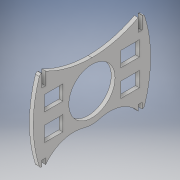
# Autodesk Inventor part: Cuerpo - Unión Laterales
Saved by Autodesk Inventor 2019 (Build 230136000, 136)
## iProperties
Created: 2020-02-15
Part Number: Cuerpo - Unión Laterales
Material: Genérico
Document SubType Name: Chapa
Designer: Mafer1
Density: 1 g/cm^3
Appearance: Valor por defecto
Sheet Metal Rule: Default
Mass: 19.1194 g
Surface Area: 143.282 cm^2
Volume: 19.1194 cm^3
soporte: 60.000 mm
largo_base: 200.000 mm
ancho_base: 80.000 mm
Author: Mafer1
Autodesk Inventor part; units mm, degrees
ref_plane "YZ Plane" through (0, 0, 0) normal (1, 0, 0) x (0, 1, 0)
ref_plane "XZ Plane" through (0, 0, 0) normal (0, 1, 0) x (-1, 0, 0)
ref_plane "XY Plane" through (0, 0, 0) normal (0, 0, 1) x (1, 0, 0)
sketch "Boceto1" plane through (0, 0, 0) normal (1, 0, 0) x (0, 1, 0)
  circle A0 centre (0, 0) radius 25
  line L0 (35, 43.5516) -> (35, 40)
  line L1 (-35, 43.5516) -> (-35, 40)
  line L2 (35, -40) -> (35, -43.5516)
  line L3 (-35, -40) -> (-35, -43.5516)
  arc A1 (33.6111, 45.4559) -> (-33.6111, 45.4559) centre (0, -59.2833) ccw
  arc A2 (-33.6111, -45.4559) -> (33.6111, -45.4559) centre (0, 59.2833) ccw
  arc A3 (-24.0379, 6.8686) -> (-35, 40) centre (-53.845, 15.3856) ccw
  arc A4 (-35, -40) -> (-24.0379, -6.8686) centre (-53.845, -15.3856) ccw
  arc A5 (35, 40) -> (24.9998, -0.1114) centre (111.9989, -0.499) ccw
  arc A6 (24.9998, 0.1114) -> (35, -40) centre (111.9989, 0.499) ccw
  arc A7 (35, 43.5516) -> (33.6111, 45.4559) centre (33, 43.5516) ccw
  arc A8 (-33.6111, 45.4559) -> (-35, 43.5516) centre (-33, 43.5516) ccw
  arc A9 (33.6111, -45.4559) -> (35, -43.5516) centre (33, -43.5516) ccw
  arc A10 (-35, -43.5516) -> (-33.6111, -45.4559) centre (-33, -43.5516) ccw
  point P0 (35, 45)
  point P1 (-35, 45)
  point P2 (35, -45)
  point P3 (-35, -45)
  dimension "d0" = 50
  dimension "d1" = 5
  dimension "d2" = 70
  dimension "d3" = 35
  dimension "d4" = 0
  dimension "d5" = 70
  dimension "d6" = 0
  dimension "d8" = 40
  dimension "d9" = 40
  dimension "d10" = 110
  dimension "d12" = 110
  dimension "d13" = 31
  dimension "d14" = 31
  dimension "d15" = 87
  dimension "d17" = 87
  dimension "d20" = 2
  dimension "d21" = 2
  dimension "d22" = 2
  constraints: 28 point on circle, 12 tangent, 11 centre point, 8 end point, 4 point on line, 4 vertical, 3 equal length, 1 coincident, 1 collinear, 1 equal radius
  measures "d0" diameter of A0
  measures "d1" distance of point (35, 45) L0.end
  measures "d2" distance between parallel lines of L1 L0
  measures "d3" distance from line of L1 point (0, 0)
  measures "d4" vertical distance of point (-35, 45) point (35, 45)
  measures "d5" distance between parallel lines of L3 L2
  measures "d6" vertical distance of point (-35, -45) point (35, -45)
  measures "d8" vertical distance of point (0, 0) L0.end
  measures "d9" vertical distance of L2.start point (0, 0)
  measures "d10" radius of A1
  measures "d12" radius of A2
  measures "d13" radius of A3
  measures "d14" radius of A4
  measures "d15" radius of A5
  measures "d17" radius of A6
  measures "d20" radius of A7
  measures "d21" radius of A9
  measures "d22" radius of A10
extrude "Extrusión1" add sketch "Boceto1" along normal blind 3.3
sketch "Boceto2" plane through (3.3, 0, 0) normal (1, 0, 0) x (0, 0, -1)
  arc A0 (-40, 35) -> (0, 25.0003) centre (0.499, 111.9989) ccw projected
  arc A1 (40, -35) -> (6.8686, -24.0379) centre (15.3856, -53.845) ccw projected
  arc A2 (0, 25.0003) -> (40, 35) centre (-0.499, 111.9989) ccw projected
  arc A3 (-6.8686, -24.0379) -> (-40, -35) centre (-15.3856, -53.845) ccw projected
  line L0 (-40, 35) -> (-43.3, 35)
  line L1 (-43.3, 35) -> (-43.3, 24)
  line L2 (-43.3, 24) -> (-40, 24)
  line L3 (-40, 24) -> (-40, 35)
  line L4 (-40, -35) -> (-43.3, -35)
  line L5 (-43.3, -35) -> (-43.3, -30)
  line L6 (-43.3, -30) -> (-40, -30)
  line L7 (-40, -30) -> (-40, -35)
  line L8 (40, 35) -> (43.3, 35)
  line L9 (43.3, 35) -> (43.3, 24)
  line L10 (43.3, 24) -> (40, 24)
  line L11 (40, 24) -> (40, 35)
  line L12 (40, -35) -> (43.3, -35)
  line L13 (43.3, -35) -> (43.3, -30)
  line L14 (43.3, -30) -> (40, -30)
  line L15 (40, -30) -> (40, -35)
  circle A4 centre (0, 0) radius 20
  line L16 (-41, 18) -> (-25, 18)
  line L17 (-25, 18) -> (-25, 5)
  line L18 (-25, 5) -> (-41, 5)
  line L19 (-41, 5) -> (-41, 18)
  line L20 (-41, -5) -> (-25, -5)
  line L21 (-25, -5) -> (-25, -18)
  line L22 (-25, -18) -> (-41, -18)
  line L23 (-41, -18) -> (-41, -5)
  line L24 (25, 18) -> (41, 18)
  line L25 (41, 18) -> (41, 5)
  line L26 (41, 5) -> (25, 5)
  line L27 (25, 5) -> (25, 18)
  line L28 (25, -5) -> (41, -5)
  line L29 (41, -5) -> (41, -18)
  line L30 (41, -18) -> (25, -18)
  line L31 (25, -18) -> (25, -5)
  point P0 (-6.2262, 34.4418)
  point P1 (12.6899, -32.6185)
  point P2 (6.2262, 34.4418)
  dimension "d31" = 40
  dimension "d23" = 3.3
  dimension "d24" = 3.3
  dimension "d25" = 3.3
  dimension "d26" = 3.3
  dimension "d27" = 11
  dimension "d28" = 5
  dimension "d34" = 16
  dimension "d35" = 13
  dimension "d37" = 25
  dimension "d38" = 5
  dimension "d40" = 5
  dimension "d41" = 25
  constraints: 64 end point, 16 parallel, 8 horizontal, 8 perpendicular, 8 point on line, 6 equal length, 1 coincident, 5 other
  measures "d23" distance of L1.end L2.end
  measures "d24" distance of L5.end L6.end
  measures "d25" distance of L13.end L14.end
  measures "d26" distance of L9.end L10.end
  measures "d27" distance of L0.end L1.end
  measures "d28" distance of L4.end L5.end
  measures "d34" distance of L16.start L16.end
  measures "d35" distance of L16.end L17.end
  measures "d37" distance from line of point (0, 0) L17
  measures "d38" distance from line of point (0, 0) L18
  measures "d40" distance from line of point (0, 0) L20
  measures "d41" distance from line of L27 point (0, 0)
extrude "Extrusión2" cut sketch "Boceto2" against normal blind 3.3
equation "\"d3\" = 0.5 * d2"
equation "\"d5\" = d2"
equation "\"d8\" = 0.5 * ancho_base"
equation "\"d9\" = d8"
equation "\"d12\" = d10"
equation "\"d14\" = d13"
equation "\"d17\" = d15"
equation "\"d25\" = d23"
equation "\"d41\" = d37"
equation "\"Radio_pliegue\" = Grosor"
equation "\"Anchura_desahogo_plegado\" = Grosor"
equation "\"Profundidad_desahogo_plegado\" = 0.5 * Grosor"
equation "\"Tamaño_destalonado\" = 4 * Grosor"
equation "\"Remanente_mínimo\" = 2 * Grosor"
equation "\"Radiodetransición\" = Radio_pliegue"
equation "\"Tamaño_de_radio_de_Jacobi\" = Grosor"
equation "\"TamañoSeparación\" = Grosor"
equation "\"Grosor\" = 0.5"
equation "\"ancho_base\" = 80"
